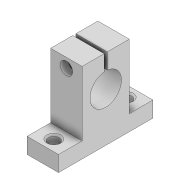
# Autodesk Inventor part: SK20
Saved by Autodesk Inventor 2020 (Build 240168000, 168)
## iProperties
Created: 2021-10-09
Part Number: SK20
Material: Generic
Document SubType Name: Modeling
Designer: Henry Cawley
Density: 1 g/cm^3
Appearance: Default
Author: Henry Cawley
Autodesk Inventor part; units mm, degrees
ref_plane "YZ Plane" through (0, 0, 0) normal (1, 0, 0) x (0, 1, 0)
ref_plane "XZ Plane" through (0, 0, 0) normal (0, 1, 0) x (-1, 0, 0)
ref_plane "XY Plane" through (0, 0, 0) normal (0, 0, 1) x (1, 0, 0)
sketch "Sketch1" plane through (0, 0, 0) normal (1, 0, 0) x (0, 1, 0)
  line L0 (0, 0) -> (0, -60)
  line L1 (0, -60) -> (10, -60)
  line L2 (10, -60) -> (10, -45)
  line L3 (10, -45) -> (51, -45)
  line L4 (51, -45) -> (51, -15)
  line L5 (51, -15) -> (10, -15)
  line L6 (10, -15) -> (10, 0)
  line L7 (10, 0) -> (0, 0)
  circle A0 centre (31, -30) radius 10
  dimension "d0" = 10
  dimension "d1" = 60
  dimension "d2" = 15
  dimension "d3" = 15
  dimension "d4" = 51
  dimension "d5" = 20
  dimension "d6" = 20
  dimension "d7" = 15
  constraints: 16 end point, 6 perpendicular, 2 point on line, 1 centre point, 1 vertical
  measures "d0" distance of L6.end L0.start
  measures "d1" distance of L0.start L0.end
  measures "d2" distance of L5.end L6.end
  measures "d3" distance of L1.end L2.end
  measures "d4" distance between parallel lines of L0 L4
  measures "d5" diameter of A0
  measures "d6" distance from line of L4 A0.centre
  measures "d7" distance from line of L5 A0.centre
extrude "Extrusion1" add sketch "Sketch1" along normal blind 20
sketch "Sketch2" plane through (20, 0, 0) normal (1, 0, 0) x (0, 0, -1)
  line L0 (45, 51) -> (15, 51) projected
  line L1 (29, 51) -> (31, 51)
  line L2 (31, 51) -> (31, 33.6332)
  line L3 (31, 33.6332) -> (29, 33.6332)
  line L4 (29, 33.6332) -> (29, 51)
  line L5 (15, 51) -> (15, 10) projected
  point P0 (0, 0)
  dimension "d10" = 2
  dimension "d12" = 14
  constraints: 8 end point, 2 parallel, 1 horizontal, 1 perpendicular, 1 point on line
  measures "d10" distance of L2.end L3.end
  measures "d12" distance between parallel lines of L5 L4
extrude "Extrusion2" cut sketch "Sketch2" against normal blind 33.25
sketch "Sketch3" plane through (0, 10, -15) normal (0, 0, 1) x (1, 0, 0)
  circle A0 centre (10, 35) radius 2.5
  line L0 (0, 41) -> (20, 41) projected
  line L1 (0, 41) -> (0, 0) projected
  point P0 (0, -10)
  dimension "d15" = 6
  dimension "d16" = 10
  dimension "d17" = 5
  constraints: 1 centre point
  measures "d15" distance from line of L0 A0.centre
  measures "d16" distance from line of L1 A0.centre
  measures "d17" diameter of A0
extrude "Extrusion3" cut sketch "Sketch3" against normal blind 33.25
sketch "Sketch4" plane through (0, 10, 0) normal (0, 1, 0) x (1, 0, 0)
  circle A0 centre (10, 7) radius 3.5
  circle A1 centre (10, 53) radius 3.5
  line L0 (20, 15) -> (20, 0) projected
  line L1 (20, 60) -> (20, 45) projected
  line L2 (0, 0) -> (20, 0) projected
  line L3 (0, 60) -> (20, 60) projected
  dimension "d20" = 7
  dimension "d21" = 10
  dimension "d22" = 10
  dimension "d23" = 7
  dimension "d24" = 7
  constraints: 2 centre point, 1 equal radius
  measures "d20" diameter of A0
  measures "d21" distance from line of L0 A0.centre
  measures "d22" distance from line of L1 A1.centre
  measures "d23" distance from line of L2 A0.centre
  measures "d24" distance from line of L3 A1.centre
extrude "Extrusion4" cut sketch "Sketch4" against normal blind 33.25
chamfer "Chamfer1" distance 1 angle 45 2 edges at (6.5, 10, -7) (6.5, 10, -53)
sketch "Sketch5" plane through (0, 10, -15) normal (0, 0, 1) x (1, 0, 0)
  circle A0 centre (10, 35) radius 2.5 projected
  circle A1 centre (10, 35) radius 4
  point P0 (0, -10)
  dimension "d30" = 8
  constraints: 1 centre point, 1 coincident
  measures "d30" diameter of A1
extrude "Extrusion5" cut sketch "Sketch5" against normal blind 5
thread "Thread1" size "M4x0.7" class "6H" standard "ANSI Metric M Profile" length 10
body "Solid1"
